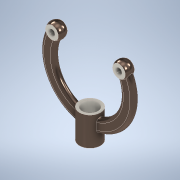
# Autodesk Inventor part: Part001.Fork
Saved by Autodesk Inventor 2022.2 (Build 262287010, 287A)
## iProperties
Created: 2022-11-28
Part Number: Part001.Fork
Material: Stainless Steel
Document SubType Name: Modeling
Designer: User
Density: 8 g/cm^3
Appearance: Gunmetal - Antique Polished
Author: User
Autodesk Inventor part; units mm, degrees
ref_plane "YZ Plane" through (0, 0, 0) normal (1, 0, 0) x (0, 1, 0)
sketch "Sketch1" plane through (0, 0, 0) normal (0, 0, 1) x (1, 0, 0)
  arc A0 (-51.303, 33) -> (51.303, 33) centre (0, 0) ccw
  line L0 (-51.303, 33) -> (51.303, 33) construction
  dimension "d0" = 122
  dimension "d1" = 33
  constraints: 2 end point, 2 point on circle, 1 centre point, 1 coincident, 1 horizontal
  measures "d0" diameter of A0
  measures "d1" distance from line of A0.centre L0
ref_plane "Work Plane1" through (-51.303, 33, 0) normal (-0.541, -0.841, 0) x (0.841, -0.541, 0)
sketch "Sketch2" plane through (-51.303, 33, 0) normal (-0.541, -0.841, 0) x (0.841, -0.541, 0)
  line L0 (-5, 0) -> (5, 0) construction
  line L1 (-5, 5) -> (5, 5)
  line L2 (5, -5) -> (-5, -5)
  arc A0 (-5, 5) -> (-5, -5) centre (-5, 0) ccw
  arc A1 (5, -5) -> (5, 5) centre (5, 0) ccw
  point P0 (61, 0)
  point P1 (0, 0)
  point P2 (0, 0)
  dimension "d2" = 10
  dimension "d3" = 5
  constraints: 8 end point, 4 point on circle, 4 tangent, 2 centre point, 1 coincident, 1 horizontal, 1 midpoint, 1 parallel
  measures "d2" distance of L2.start L2.end
  measures "d3" radius of A1
sweep "Sweep1" add profiles "Sketch2" path "Sketch1"
sketch "Sketch3" plane through (-51.303, 33, 0) normal (-0.541, -0.841, 0) x (0.841, -0.541, 0)
  line L0 (0, 7) -> (9.7468, 7)
  line L1 (9.7468, -7) -> (0, -7)
  line L2 (0, -7) -> (0, 7)
  arc A0 (9.7468, -7) -> (9.7468, 7) centre (0, 0) ccw
  line L3 (5, 5) -> (-5, 5) construction
  arc A1 (5, -5) -> (5, 5) centre (5, 0) ccw construction
  line L4 (-5, -5) -> (5, -5) construction
  arc A2 (-5, 5) -> (-5, -5) centre (-5, 0) ccw construction
  line L5 (-5, -5) -> (5, -5) projected
  point P0 (61, 0)
  point P1 (0, -5)
  dimension "d6" = 14
  dimension "d7" = 12
  constraints: 6 end point, 2 midpoint, 2 point on circle, 1 centre point, 1 coincident, 1 horizontal, 1 horizontal alignment, 1 parallel, 1 perpendicular, 1 point on line
  measures "d6" distance of L0.start L1.end
  measures "d7" radius of A0
revolve "Revolution1" add sketch "Sketch3" angle 360 about axis through (-51.303, 33, -7) along (0, 0, 1)
sketch "Sketch4" plane through (-51.303, 33, 7) normal (0, 0, 1) x (1, 0, 0)
  circle A0 centre (0, 0) radius 9.7468 projected
  point P0 (51.303, -33)
  constraints: 1 coincident
hole "Hole1" at (-51.303, 33, 7) direction (0, 0, -1) diameter 9 end through all
mirror "Mirror1" about plane through (0, 0, 0) normal (1, 0, 0) of "Revolution1", "Hole1"
ref_plane "Work Plane2" through (0, -87, 0) normal (0, 1, 0) x (-1, 0, 0)
sketch "Sketch5" plane through (0, -87, 0) normal (0, 1, 0) x (-1, 0, 0)
  circle A0 centre (0, 0) radius 16
  dimension "d17" = 32
  constraints: 1 centre point, 1 coincident
  measures "d17" diameter of A0
extrude "Extrusion1" add sketch "Sketch5" along normal blind 44
sketch "Sketch6" plane through (0, -43, 0) normal (0, 1, 0) x (1, 0, 0)
  circle A0 centre (0, 0) radius 16 projected
  constraints: 1 coincident
hole "Hole2" at (0, -43, 0) direction (0, -1, 0) diameter 24 end through all
sketch "Sketch7" plane through (0, 0, 0) normal (0, 0, 1) x (1, 0, 0)
  line L0 (-12, -87) -> (-12, -43) construction
  line L1 (0, -113.4) -> (0, 71.4) projected
  line L2 (-12, -81) -> (-14, -81)
  line L3 (-14, -81) -> (-14, -83)
  line L4 (-14, -83) -> (-12, -83)
  line L5 (-12, -83) -> (-12, -81)
  line L6 (16, -87) -> (-16, -87) construction
  point P0 (0, 0)
  dimension "d27" = 2
  dimension "d28" = 28
  dimension "d29" = 6
  constraints: 8 end point, 2 parallel, 1 collinear, 1 horizontal, 1 perpendicular
  measures "d27" distance of L3.end L2.end
  measures "d28" diameter of L3 L1
  measures "d29" distance from line of L6 L2.end
revolve "Revolution2" cut sketch "Sketch7" angle 360 about axis through (0, -10, 0) along (0, -1, 0)
body "Solid1"
